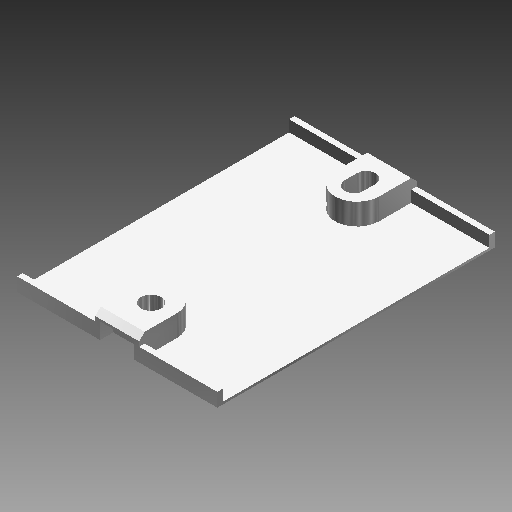
# Autodesk Inventor part: SSR-40 DA BOTTOM
Saved by Autodesk Inventor 2019 (Build 230136000, 136)
## iProperties
Created: 2014-10-30
Part Number: SSR-40 DA BOTTOM
Material: Nickel-Copper Alloy 400
Document SubType Name: Modeling
Designer: Tyler
Density: 8.83 g/cm^3
Appearance: Chrome - Polished
Mass: 21.9457 g
Surface Area: 65.9663 cm^2
Volume: 2.48536 cm^3
Author: Tyler
Autodesk Inventor part; units mm, degrees
ref_plane "YZ Plane" through (0, 0, 0) normal (1, 0, 0) x (0, 1, 0)
ref_plane "XZ Plane" through (0, 0, 0) normal (0, 1, 0) x (-1, 0, 0)
ref_plane "XY Plane" through (0, 0, 0) normal (0, 0, 1) x (1, 0, 0)
sketch "Sketch1" plane through (0, 0, 0) normal (0, 1, 0) x (-1, 0, 0)
  line L0 (22.4663, 31.1531) -> (-22.4663, 31.1531)
  line L1 (-22.4663, 31.1531) -> (-22.4663, -31.1531)
  line L2 (-22.4663, -31.1531) -> (22.4663, -31.1531)
  line L3 (22.4663, -31.1531) -> (22.4663, 31.1531)
  point P0 (0, 0)
  point P1 (22.4663, 0)
  point P2 (0, -31.1531)
  dimension "d0" = 62.3062
  dimension "d1" = 44.9326
  constraints: 8 end point, 2 midpoint, 2 parallel, 1 horizontal, 1 horizontal alignment, 1 perpendicular, 1 vertical alignment
  measures "d0" distance of L1.end L0.end
  measures "d1" distance of L0.start L0.end
extrude "Extrusion1" add sketch "Sketch1" along normal blind 0.5334
sketch "Sketch2" plane through (0, 0.5334, 0) normal (0, 1, 0) x (1, 0, 0)
  line L0 (22.4663, -31.1531) -> (22.4663, 31.1531) projected
  line L1 (-22.4663, 31.1531) -> (22.4663, 31.1531)
  line L2 (22.4663, 31.1531) -> (22.4663, 29.9085)
  line L3 (22.4663, 29.9085) -> (-22.4663, 29.9085)
  line L4 (-22.4663, 29.9085) -> (-22.4663, 31.1531)
  line L5 (-22.4663, -31.1531) -> (22.4663, -31.1531)
  line L6 (22.4663, -31.1531) -> (22.4663, -29.9085)
  line L7 (22.4663, -29.9085) -> (-22.4663, -29.9085)
  line L8 (-22.4663, -29.9085) -> (-22.4663, -31.1531)
  line L9 (-22.4663, -31.1531) -> (22.4663, -31.1531) projected
  point P0 (0, 0)
  dimension "d4" = 1.2446
  dimension "d5" = 1.2446
  dimension "d6" = 59.817
  dimension "d7" = 0
  constraints: 16 end point, 4 parallel, 2 horizontal, 2 perpendicular, 2 point on line
  measures "d4" distance between parallel lines of L3 L1
  measures "d5" distance between parallel lines of L5 L7
  measures "d6" distance between parallel lines of L7 L3
  measures "d7" distance between parallel lines of L9 L5
extrude "Extrusion2" add sketch "Sketch2" along normal blind 2.54
sketch "Sketch3" plane through (0, 0.5334, 0) normal (0, 1, 0) x (1, 0, 0)
  line L0 (22.4663, 29.9085) -> (-22.4663, 29.9085) projected
  line L1 (4.9276, 29.9085) -> (-4.9276, 29.9085)
  line L2 (-4.9276, 29.9085) -> (-4.9276, 22.6949)
  line L3 (0, 17.7673) -> (0, 17.7673)
  line L4 (4.9276, 22.6949) -> (4.9276, 29.9085)
  arc A0 (-4.9276, 22.6949) -> (0, 17.7673) centre (0, 22.6949) ccw
  arc A1 (0, 17.7673) -> (4.9276, 22.6949) centre (0, 22.6949) ccw
  line L5 (22.4663, -29.9085) -> (-22.4663, -29.9085) projected
  line L6 (4.9276, -29.9085) -> (-4.9276, -29.9085)
  line L7 (-4.9276, -29.9085) -> (-4.9276, -22.6949)
  line L8 (0, -17.7673) -> (0, -17.7673)
  line L9 (4.9276, -22.6949) -> (4.9276, -29.9085)
  arc A2 (4.9276, -22.6949) -> (0, -17.7673) centre (0, -22.6949) ccw
  arc A3 (0, -17.7673) -> (-4.9276, -22.6949) centre (0, -22.6949) ccw
  point P0 (0, 0)
  point P1 (-4.9276, 17.7673)
  point P2 (4.9276, 17.7673)
  point P3 (0, 17.7673)
  point P4 (-4.9276, -17.7673)
  point P5 (4.9276, -17.7673)
  dimension "d10" = 12.1412
  dimension "d11" = 9.8552
  dimension "d12" = 4.9276
  dimension "d13" = 9.8552
  dimension "d14" = 12.1412
  dimension "d15" = 4.9276
  dimension "d16" = 4.9276
  constraints: 16 end point, 10 point on line, 8 point on circle, 8 tangent, 4 centre point, 4 parallel, 2 horizontal, 2 perpendicular, 1 concentric, 1 midpoint, 1 vertical alignment
  measures "d10" distance of point (-4.928, 17.767) L1.end
  measures "d11" distance of point (-4.928, 17.767) point (4.928, 17.767)
  measures "d12" radius of A0
  measures "d13" distance of point (-4.928, -17.767) point (4.928, -17.767)
  measures "d14" distance of L6.end point (-4.928, -17.767)
  measures "d15" radius of A2
  measures "d16" radius of A3
extrude "Extrusion3" add sketch "Sketch3" along normal blind 4.826
sketch "Sketch4" plane through (0, 3.0734, 0) normal (0, 1, 0) x (1, 0, 0)
  line L0 (-22.4663, -31.1531) -> (22.4663, -31.1531) projected
  line L1 (4.9276, -29.9085) -> (-4.9276, -29.9085)
  line L2 (-4.9276, -29.9085) -> (-4.9276, -31.1531)
  line L3 (-4.9276, -31.1531) -> (4.9276, -31.1531)
  line L4 (4.9276, -31.1531) -> (4.9276, -29.9085)
  line L5 (22.4663, 31.1531) -> (-22.4663, 31.1531) projected
  line L6 (4.9276, 29.9085) -> (-4.9276, 29.9085)
  line L7 (-4.9276, 29.9085) -> (-4.9276, 31.1531)
  line L8 (-4.9276, 31.1531) -> (4.9276, 31.1531)
  line L9 (4.9276, 31.1531) -> (4.9276, 29.9085)
  point P0 (0, 0)
  constraints: 16 end point, 4 parallel, 3 point on line, 2 horizontal, 2 perpendicular
extrude "Extrusion4" add sketch "Sketch4" along normal blind 2.286
chamfer "Chamfer1" distance 1.2446 angle 45 2 edges at (0, 5.3594, 31.1531) (0, 5.3594, -31.1531)
sketch "Sketch5" plane through (0, 0, 0) normal (0, -1, 0) x (1, 0, 0)
  line L0 (22.4663, -31.1531) -> (-22.4663, -31.1531) projected
  line L1 (-3.8481, -31.1531) -> (3.8481, -31.1531)
  line L2 (3.8481, -31.1531) -> (3.8481, -28.1813)
  line L3 (3.8481, -28.1813) -> (-3.8481, -28.1813)
  line L4 (-3.8481, -28.1813) -> (-3.8481, -31.1531)
  line L5 (-22.4663, 31.1531) -> (22.4663, 31.1531) projected
  line L6 (-3.8481, 31.1531) -> (3.8481, 31.1531)
  line L7 (3.8481, 31.1531) -> (3.8481, 28.1813)
  line L8 (3.8481, 28.1813) -> (-3.8481, 28.1813)
  line L9 (-3.8481, 28.1813) -> (-3.8481, 31.1531)
  point P0 (0, 0)
  point P1 (0, -31.1531)
  point P2 (0, -28.1813)
  point P3 (0, 28.1813)
  point P4 (0, 31.1531)
  dimension "d24" = 7.6962
  dimension "d25" = 2.9718
  dimension "d26" = 2.9718
  constraints: 16 end point, 4 midpoint, 4 parallel, 2 horizontal, 2 perpendicular, 2 point on line, 2 vertical alignment
  measures "d24" distance of L3.end L2.end
  measures "d25" distance of L2.end L1.end
  measures "d26" distance of L6.end L7.end
extrude "Extrusion5" cut sketch "Sketch5" against normal blind 3.6068
sketch "Sketch6" plane through (0, 5.3594, 0) normal (0, 1, 0) x (1, 0, 0)
  line L0 (0, 19.9009) -> (0, 19.9009)
  line L1 (2.0955, 21.9964) -> (2.0955, 24.765)
  line L2 (0, 26.8605) -> (0, 26.8605)
  line L3 (-2.0955, 24.765) -> (-2.0955, 21.9964)
  line L4 (4.9276, 31.1531) -> (-4.9276, 31.1531) projected
  arc A0 (0, 19.9009) -> (2.0955, 21.9964) centre (0, 21.9964) ccw
  arc A1 (-2.0955, 21.9964) -> (0, 19.9009) centre (0, 21.9964) ccw
  arc A2 (0, 26.8605) -> (-2.0955, 24.765) centre (0, 24.765) ccw
  arc A3 (2.0955, 24.765) -> (0, 26.8605) centre (0, 24.765) ccw
  circle A4 centre (0, -23.5331) radius 2.2606
  line L5 (-4.9276, -31.1531) -> (4.9276, -31.1531) projected
  point P0 (0, 0)
  point P1 (2.0955, 26.8605)
  point P2 (2.0955, 19.9009)
  point P3 (-2.0955, 26.8605)
  point P4 (0, 19.9009)
  dimension "d29" = 4.191
  dimension "d30" = 6.9596
  dimension "d31" = 4.2926
  dimension "d32" = 2.0955
  dimension "d33" = 2.0955
  dimension "d34" = 2.0955
  dimension "d35" = 7.62
  dimension "d38" = 4.5212
  constraints: 8 end point, 8 point on circle, 8 tangent, 6 point on line, 5 centre point, 2 parallel, 2 vertical alignment, 1 concentric, 1 horizontal, 1 midpoint, 1 perpendicular
  measures "d29" distance of point (-2.096, 26.86) point (2.096, 26.86)
  measures "d30" distance of point (2.096, 26.86) point (2.095, 19.901)
  measures "d31" distance between parallel lines of L4 L2
  measures "d32" radius of A0
  measures "d33" radius of A2
  measures "d34" radius of A3
  measures "d35" distance from line of L5 A4.centre
  measures "d38" diameter of A4
extrude "Extrusion6" cut sketch "Sketch6" against normal through all
body "Solid1"
